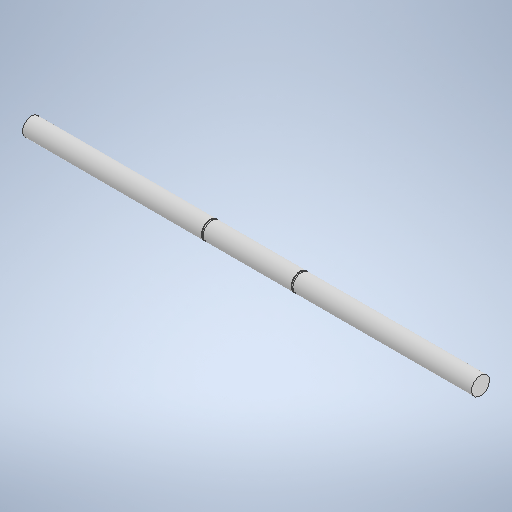
# Autodesk Inventor part: Part2
Saved by Autodesk Inventor 2025.2 (Build 292293000, 293)
## iProperties
Created: 2025-01-12
Part Number: Part2
Material: Generic
Document SubType Name: Modeling
Designer: caomi
Density: 1 g/cm^3
Appearance: Default
Author: caomi
Autodesk Inventor part; units mm, degrees
ref_plane "XZ Plane" through (0, 0, 0) normal (0, 1, 0) x (-1, 0, 0)
ref_plane "XY Plane" through (0, 0, 0) normal (0, 0, 1) x (1, 0, 0)
sketch "Sketch1" plane through (0, 0, 0) normal (1, 0, 0) x (0, 1, 0)
  circle A0 centre (0, 0) radius 2.5
  circle A1 centre (0, 0) radius 2.3
  dimension "d0" = 5
  dimension "d3" = 0.2
  constraints: 2 centre point, 1 coincident
  measures "d0" diameter of A0
  measures "d3" radial gap between concentric circles of A1 A0
extrude "Extrusion1" add sketch "Sketch1" along normal mid plane 125 contours A0 | A1
ref_plane "Work Plane1" through (12.5, 0, 0) normal (1, 0, 0) x (0, 1, 0)
extrude "Extrusion3" cut sketch "Sketch1" along normal mid plane 0.5 from surface at 12.5
mirror "Mirror1" about plane through (0, 0, 0) normal (1, 0, 0) of "Extrusion3"
body "Solid1"
